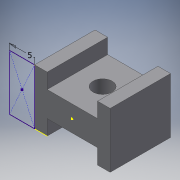
# Autodesk Inventor part: StopRotation
Saved by Autodesk Inventor 2019 (Build 230136000, 136)
## iProperties
Created: 2019-08-02
Part Number: StopRotation
Material: Generic
Document SubType Name: Modeling
Designer: aorfi
Density: 1 g/cm^3
Appearance: Default
Author: aorfi
Autodesk Inventor part; units mm, degrees
ref_plane "YZ Plane" through (0, 0, 0) normal (1, 0, 0) x (0, 1, 0)
ref_plane "XZ Plane" through (0, 0, 0) normal (0, 1, 0) x (-1, 0, 0)
ref_plane "XY Plane" through (0, 0, 0) normal (0, 0, 1) x (1, 0, 0)
sketch "Sketch1" plane through (0, 0, 0) normal (0, 1, 0) x (-1, 0, 0)
  line L0 (-7.5, 6) -> (7.5, 6)
  line L1 (7.5, 6) -> (7.5, -6)
  line L2 (7.5, -6) -> (-7.5, -6)
  line L3 (-7.5, -6) -> (-7.5, 6)
  line L4 (-7.5, 6) -> (7.5, -6) construction
  line L5 (7.5, 6) -> (-7.5, -6) construction
  point P0 (0, 0)
  dimension "d0" = 12
  dimension "d1" = 15
  constraints: 12 end point, 2 midpoint, 2 parallel, 1 horizontal, 1 perpendicular
  measures "d0" distance of L0.end L1.end
  measures "d1" distance of L1.end L2.end
extrude "Extrusion1" add sketch "Sketch1" along normal mid plane 5
sketch "Sketch2" plane through (0, 2.5, 0) normal (0, 1, 0) x (1, 0, 0)
  line L0 (-5, 6) -> (-7.5, 6)
  line L1 (-7.5, 6) -> (-7.5, -6)
  line L2 (-7.5, -6) -> (-5, -6)
  line L3 (-5, -6) -> (-5, 6)
  line L4 (-5, 6) -> (-7.5, -6) construction
  line L5 (-7.5, 6) -> (-5, -6) construction
  line L6 (7.5, -6) -> (7.5, 6) projected
  line L7 (5, 6) -> (7.5, 6)
  line L8 (7.5, 6) -> (7.5, -6)
  line L9 (7.5, -6) -> (5, -6)
  line L10 (5, -6) -> (5, 6)
  line L11 (5, 6) -> (7.5, -6) construction
  line L12 (7.5, 6) -> (5, -6) construction
  line L13 (5, 0) -> (-5, 0) construction
  point P0 (0, 0)
  point P1 (-6.25, 0)
  point P2 (6.25, 0)
  point P3 (0, 0)
  dimension "d15" = 10
  constraints: 26 end point, 7 midpoint, 4 parallel, 2 coincident, 2 horizontal, 2 perpendicular, 1 point on line
  measures "d15" distance between parallel lines of L3 L10
extrude "Extrusion2" add sketch "Sketch2" along normal blind 3
sketch "Sketch3" plane through (0, -2.5, 0) normal (0, -1, 0) x (1, 0, 0)
  point P0 (0, 0)
hole "Hole1" at (0, -2.5, 0) direction (0, 1, 0) diameter 3.797 end through all clearance for "Flat Head Machine Screw (82)" size "#6" standard "Ansi Unified Screw Threads"
mirror "Mirror1" about plane through (0, 0, 0) normal (0, 1, 0)
sketch "Sketch4" plane through (-5, 2.5, 6) normal (0, 0, 1) x (1, 0, 0)
  line L0 (-2.5, 3) -> (-2.5, -8) projected
  line L1 (-10.5, -8) -> (-2.5, -8)
  line L2 (-2.5, -8) -> (-2.5, 3)
  line L3 (-2.5, 3) -> (-10.5, 3)
  line L4 (-10.5, 3) -> (-10.5, -8)
  line L5 (-10.5, -8) -> (-2.5, 3) construction
  line L6 (-2.5, -8) -> (-10.5, 3) construction
  line L7 (-2.5, -8) -> (0, -8) projected
  point P0 (5, -2.5)
  point P1 (-6.5, -2.5)
  dimension "d16" = 8
  constraints: 12 end point, 2 midpoint, 2 parallel, 1 collinear, 1 horizontal, 1 perpendicular
  measures "d16" distance between parallel lines of L0 L4
extrude "Extrusion3" add sketch "Sketch4" against normal blind 5
sketch "Sketch5" plane through (-5, 2.5, 1) normal (0, 0, -1) x (-1, 0, 0)
  line L0 (10.5, -8) -> (10.5, 3) projected
  line L1 (2.5, -8) -> (10.5, -8) projected
  circle A0 centre (6.5, -2.5) radius 2.55
  point P0 (-5, -2.5)
  point P1 (10.5, -2.5)
  point P2 (6.5, -8)
  point P3 (10.5, -2.5)
  point P4 (6.5, -8)
  point P5 (6.5, -8)
  dimension "d19" = 5.1
  constraints: 5 midpoint, 1 centre point, 1 horizontal alignment, 1 vertical alignment
  measures "d19" diameter of A0
extrude "Extrusion4" cut sketch "Sketch5" against normal through all
fillet "Fillet1" radius 2 2 edges at (-15.5, 5.5, 3.5) (-15.5, -5.5, 3.5)
body "Solid1"
